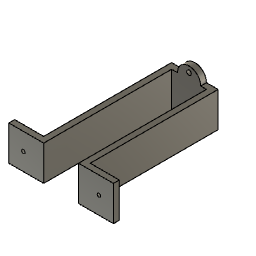
SoporteAletaAerodeslizador v1 (Autodesk Fusion 360 design; units mm, degrees)
Autodesk Fusion 360 part; units mm, degrees
note: some values were not read from the file. Set by a fixed rule: which sketch regions a step uses.
sketch "Boceto1" plane through (0, 0, 0) normal (0, 0, 1) x (1, 0, 0)
  line L0 (0, 0) -> (30, 0)
  line L1 (30, 0) -> (30, 110)
  line L2 (30, 110) -> (60, 110)
  line L3 (60, 110) -> (60, 0)
  line L4 (60, 0) -> (90, 0)
  line L5 (90, 0) -> (90, 5)
  line L6 (90, 5) -> (65, 5)
  line L7 (65, 5) -> (65, 115)
  line L8 (65, 115) -> (25, 115)
  line L9 (25, 115) -> (25, 5)
  line L10 (25, 5) -> (0, 5)
  line L11 (0, 5) -> (0, 0)
  dimension "d1" = 110
  dimension "d2" = 5
  dimension "d3" = 25
  dimension "d4" = 110
  dimension "d5" = 40
  dimension "d6" = 110
  constraint coincident L0.start L11.end
  constraint horizontal L0
  constraint perpendicular L0 L1
  constraint perpendicular L1 L2
  constraint perpendicular L2 L3
  constraint perpendicular L3 L4
  constraint perpendicular L4 L5
  constraint perpendicular L3 L6
  constraint perpendicular L2 L7
  constraint perpendicular L7 L8
  constraint perpendicular L8 L9
  constraint perpendicular L9 L10
  constraint perpendicular L0 L11
  measures "d1" distance of L0.end L1.end
  measures "d2" distance of L4.end L5.end
  measures "d3" distance of L5.end L6.end
  measures "d4" distance of L6.end L7.end
  measures "d5" distance of L7.end L8.end
  measures "d6" distance of L8.end L9.end
extrude "Extruir1" add sketch "Boceto1" along normal blind 30
sketch "Boceto2" plane through (0, 115, 0) normal (0, 1, 0) x (-1, 0, 0)
  line L0 (-65, 0) -> (-25, 0)
  line L1 (-25, 0) -> (-25, 30)
  line L2 (-25, 30) -> (-65, 30)
  line L3 (-65, 30) -> (-65, 0)
  circle A0 centre (-45, 30) radius 10
  constraint midpoint L2 A0.centre
extrude "Extruir2" add sketch "Boceto2" against normal blind 5 contours L2 A0 picked at (-42.135, 33.3571)
sketch "Boceto3" plane through (0, 115, 0) normal (0, 1, 0) x (-1, 0, 0)
  line L0 (-65, 0) -> (-25, 0)
  line L1 (-25, 0) -> (-25, 30)
  line L2 (-25, 30) -> (-35, 30)
  arc A0 (-35, 30) -> (-55, 30) centre (-45, 30) ccw
  line L3 (-55, 30) -> (-65, 30)
  line L4 (-65, 30) -> (-65, 0)
  line L5 (-45, 40) -> (-45, 35)
  circle A1 centre (-45, 35) radius 2
  dimension "d11" = 5
  dimension "d12" = 4
  constraint midpoint A0 L5.start
  constraint vertical L5
  constraint coincident L5.end A1.centre
  measures "d11" distance of L5.start L5.end
  measures "d12" diameter of A1
extrude "Extruir3" cut sketch "Boceto3" against normal blind 5 contours A1
sketch "Boceto4" plane through (0, 5, 0) normal (0, 1, 0) x (-1, 0, 0)
  line L0 (-25, 0) -> (0, 0)
  line L1 (0, 0) -> (0, 30)
  line L2 (0, 30) -> (-25, 30)
  line L3 (-25, 30) -> (-25, 0)
  line L4 (-25, 30) -> (0, 0)
  line L5 (0, 30) -> (-25, 0)
  line L6 (-65, 0) -> (-90, 30)
  line L7 (-90, 30) -> (-90, 0)
  line L8 (-90, 0) -> (-65, 30)
  circle A0 centre (-77.5, 15) radius 1.5
  circle A1 centre (-12.5, 15) radius 1.5
  dimension "d15" = 3
  dimension "d16" = 3
  constraint coincident L2.end L3.start
  constraint coincident L0.end L1.start
  constraint coincident L1.end L2.start
  constraint coincident L0.start L3.end
  constraint parallel L4 L6
  constraint vertical L7
  constraint parallel L5 L8
  constraint midpoint L6 A0.centre
  constraint midpoint L4 A1.centre
  measures "d15" diameter of A0
  measures "d16" diameter of A1
extrude "Extruir4" cut sketch "Boceto4" against normal blind 5 contours L4 L5 A1 | L4 L5 A1 | L4 L5 A1 | L4 L5 A1 | L6 L8 A0 | L6 L8 A0 | L6 L8 A0 | L6 L8 A0
